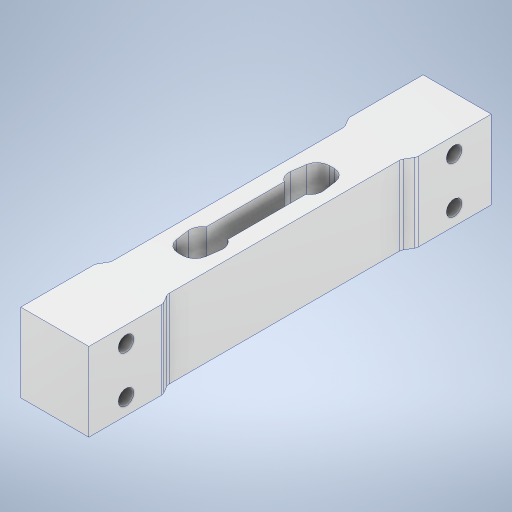
# Autodesk Inventor part: Célula de carga 3
Saved by Autodesk Inventor 2023.2 (Build 272271030, 271C)
## iProperties
Created: 2023-04-15
Part Number: Célula de carga 3
Material: Alumínio 6061
Document SubType Name: Sheet Metal
Designer: Mateus PC
Density: 2.7 g/cm^3
Sheet Metal Rule: Padrão_mm
Appearance: Alumínio - Plano
Author: Mateus PC
Autodesk Inventor part; units mm, degrees
ref_plane "YZ Plane" through (0, 0, 0) normal (1, 0, 0) x (0, 1, 0)
ref_plane "XZ Plane" through (0, 0, 0) normal (0, 1, 0) x (-1, 0, 0)
ref_plane "XY Plane" through (0, 0, 0) normal (0, 0, 1) x (1, 0, 0)
sketch "Esboço1" plane through (0, 0, 0) normal (0, 1, 0) x (-1, 0, 0)
  line L0 (0, 0) -> (22, 0)
  line L1 (22, 0) -> (22, -23.4641)
  line L2 (22, -24) -> (25.6764, -24) construction
  line L3 (0, 0) -> (0, -23.4641)
  line L4 (1.9, -27.8268) -> (1.9, -102.1732)
  line L5 (0, -106.5359) -> (0, -130)
  line L6 (0, -130) -> (22, -130)
  line L7 (22, -130) -> (22, -106.5359)
  line L8 (20.1, -102.1732) -> (20.1, -27.8268)
  line L9 (21.7321, -24.4641) -> (20.3679, -26.8268)
  line L10 (1.6321, -26.8268) -> (0.2679, -24.4641)
  line L11 (20.3679, -103.1732) -> (21.7321, -105.5359)
  line L12 (0.2679, -105.5359) -> (1.6321, -103.1732)
  arc A0 (21.7321, -24.4641) -> (22, -23.4641) centre (20, -23.4641) ccw
  arc A1 (20.3679, -26.8268) -> (20.1, -27.8268) centre (22.1, -27.8268) ccw
  arc A2 (1.9, -27.8268) -> (1.6321, -26.8268) centre (-0.1, -27.8268) ccw
  arc A3 (0, -23.4641) -> (0.2679, -24.4641) centre (2, -23.4641) ccw
  arc A4 (22, -106.5359) -> (21.7321, -105.5359) centre (20, -106.5359) ccw
  arc A5 (20.1, -102.1732) -> (20.3679, -103.1732) centre (22.1, -102.1732) ccw
  arc A6 (1.6321, -103.1732) -> (1.9, -102.1732) centre (-0.1, -102.1732) ccw
  arc A7 (0.2679, -105.5359) -> (0, -106.5359) centre (2, -106.5359) ccw
  line L13 (7.5, -52.4035) -> (7.5, -77.5965)
  spline S0 degree 3 poles (7.5, -52.4035) (7.1712, -52.2005) (6.8736, -51.9509) (6.3593, -51.374) (6.1453, -51.0498) (5.8168, -50.3503) (5.704, -49.9786) (5.5886, -49.2144) (5.5866, -48.826) (5.6404, -48.4433) knots 0 0 0 0 0.250007 0.250007 0.5 0.5 0.749993 0.749993 1 1 1 1
  line L14 (5.6404, -48.4433) -> (6.2661, -43.9914)
  spline S1 degree 3 poles (6.2661, -43.9914) (6.3326, -43.5177) (6.4837, -43.0598) (6.9401, -42.2191) (7.2419, -41.8431) (7.9639, -41.2155) (8.3783, -40.9689) (9.2743, -40.6339) (9.7488, -40.5481) (10.2271, -40.5481) knots -0.574004 -0.574004 -0.574004 -0.574004 -0.430503 -0.430503 -0.287003 -0.287003 -0.143502 -0.143502 -0.000001 -0.000001 -0.000001 -0.000001
  line L15 (10.2271, -40.5481) -> (11.7729, -40.5481)
  spline S2 degree 3 poles (11.7729, -40.5481) (12.2512, -40.5481) (12.7257, -40.6339) (13.6217, -40.9689) (14.0361, -41.2155) (14.7581, -41.8431) (15.0599, -42.2191) (15.5163, -43.0598) (15.6674, -43.5177) (15.7339, -43.9914) knots -0.574004 -0.574004 -0.574004 -0.574004 -0.430503 -0.430503 -0.287003 -0.287003 -0.143502 -0.143502 -0.000001 -0.000001 -0.000001 -0.000001
  line L16 (15.7339, -43.9914) -> (16.3596, -48.4433)
  spline S3 degree 3 poles (16.3596, -48.4433) (16.4134, -48.826) (16.4114, -49.2144) (16.296, -49.9786) (16.1832, -50.3503) (15.8547, -51.0498) (15.6407, -51.374) (15.1264, -51.9509) (14.8288, -52.2005) (14.5, -52.4035) knots 0 0 0 0 0.250007 0.250007 0.5 0.5 0.749993 0.749993 1 1 1 1
  line L17 (14.5, -77.5965) -> (14.5, -52.4035)
  spline S4 degree 3 poles (14.5, -77.5965) (14.8288, -77.7995) (15.1264, -78.0491) (15.6407, -78.626) (15.8547, -78.9502) (16.1832, -79.6497) (16.296, -80.0214) (16.4114, -80.7856) (16.4134, -81.174) (16.3596, -81.5567) knots 0 0 0 0 0.250007 0.250007 0.5 0.5 0.749993 0.749993 1 1 1 1
  line L18 (15.7339, -86.0086) -> (16.3596, -81.5567)
  spline S5 degree 3 poles (15.7339, -86.0086) (15.6674, -86.4823) (15.5163, -86.9402) (15.0599, -87.7809) (14.7581, -88.1569) (14.0361, -88.7845) (13.6217, -89.0311) (12.7257, -89.3661) (12.2512, -89.4519) (11.7729, -89.4519) knots -0.574004 -0.574004 -0.574004 -0.574004 -0.430503 -0.430503 -0.287003 -0.287003 -0.143502 -0.143502 -0.000001 -0.000001 -0.000001 -0.000001
  spline S6 degree 3 poles (10.2271, -89.4519) (9.7488, -89.4519) (9.2743, -89.3661) (8.3783, -89.0311) (7.9639, -88.7845) (7.2419, -88.1569) (6.9401, -87.7809) (6.4837, -86.9402) (6.3326, -86.4823) (6.2661, -86.0086) knots -0.574004 -0.574004 -0.574004 -0.574004 -0.430503 -0.430503 -0.287003 -0.287003 -0.143502 -0.143502 -0.000001 -0.000001 -0.000001 -0.000001
  line L19 (10.2271, -89.4519) -> (11.7729, -89.4519)
  line L20 (5.6404, -81.5567) -> (6.2661, -86.0086)
  spline S7 degree 3 poles (5.6404, -81.5567) (5.5866, -81.174) (5.5886, -80.7856) (5.704, -80.0214) (5.8168, -79.6497) (6.1453, -78.9502) (6.3593, -78.626) (6.8736, -78.0491) (7.1712, -77.7995) (7.5, -77.5965) knots 0 0 0 0 0.250007 0.250007 0.5 0.5 0.749993 0.749993 1 1 1 1
  point P0 (20.1, -27.2909)
  point P1 (0, -24)
  point P2 (1.9, -27.2909)
  point P3 (0, -106)
  point P4 (22, -106)
  point P5 (20.1, -102.7091)
  point P6 (11, -130)
  point P7 (11, -89.4519)
  point P8 (11, -40.5481)
  point P9 (20.1, -65)
  point P10 (14.5, -65)
  dimension "d0" = 22
  dimension "d1" = 24
  dimension "d4" = 3.8
  dimension "d6" = 3.8
  dimension "d7" = 24
  dimension "d8" = 18.2
  dimension "d10" = 0
  dimension "d11" = 130
  dimension "d12" = 1.9
  dimension "d13" = 2
  dimension "d14" = 2
  dimension "d38" = 7
  dimension "d39" = 7
  dimension "d40" = 4.4957
  dimension "d41" = 4.4957
  dimension "d42" = 4.4519
  dimension "d43" = 0.6257
  dimension "d44" = 172
  dimension "d45" = 1.5457
  dimension "d46" = 1.5457
  dimension "d47" = 0.6257
  dimension "d48" = 4.4519
  dimension "d49" = 3.9611
  dimension "d50" = 3.4433
  dimension "d51" = 9.4679
  dimension "d52" = 3.9611
  dimension "d53" = 3.9602
  dimension "d54" = 1.8596
  dimension "d55" = 4.4519
  dimension "d56" = 3.9602
  dimension "d57" = 3.9602
  dimension "d58" = 4.3751
  dimension "d59" = 1.8596
  dimension "d60" = 3.9611
  dimension "d61" = 3.9611
  dimension "d62" = 3.4433
  dimension "d63" = 3.4433
  dimension "d64" = 0
  dimension "d65" = 48.9038
  dimension "d67" = 0
  constraints: 42 end point, 16 point on circle, 16 point on line, 16 tangent, 8 centre point, 6 equal length, 6 equal radius, 5 midpoint, 4 horizontal, 4 vertical, 3 perpendicular, 1 parallel, 16 other
  measures "d0" distance of L0.start L0.end
  measures "d1" distance of L0.end L2.start
  measures "d4" distance of point (0, -24) point (1.9, -27.291)
  measures "d6" distance of point (22, -106) point (20.1, -102.709)
  measures "d7" distance of point (0, -106) L5.end
  measures "d8" distance between parallel lines of L4 L8
  measures "d10" vertical distance of point (1.9, -27.291) point (20.1, -27.291)
  measures "d11" distance of L6.end L0.end
  measures "d12" horizontal distance of L2.start point (20.1, -27.291)
  measures "d13" radius of A0
  measures "d14" radius of A7
  measures "d38" distance between parallel lines of L13 L17
  measures "d39" distance of L13.end L17.start
  measures "d40" distance of L16.start L16.end
  measures "d41" distance of L14.start L14.end
  measures "d42" vertical distance of L14.start L14.end
  measures "d43" horizontal distance of L14.start L14.end
  measures "d44" angle of L13 L14
  measures "d45" distance of L15.start L15.end
  measures "d46" distance of L19.start L19.end
  measures "d47" horizontal distance of L20.start L20.end
  measures "d48" vertical distance of L18.end L18.start
  measures "d49" horizontal distance of L18.start L19.end
  measures "d50" vertical distance of L19.end L18.start
  measures "d51" distance of L20.end L18.start
  measures "d52" horizontal distance of L20.end L19.start
  measures "d53" vertical distance of L20.start L13.end
  measures "d54" horizontal distance of L20.start L13.end
  measures "d55" vertical distance of L16.end L16.start
  measures "d56" vertical distance of L16.end L17.end
  measures "d57" vertical distance of L14.start L13.start
  measures "d58" distance of L13.start L14.start
  measures "d59" horizontal distance of L16.end L17.end
  measures "d60" horizontal distance of L14.end L15.start
  measures "d61" horizontal distance of L15.end L16.start
  measures "d62" vertical distance of L15.end L16.start
  measures "d63" vertical distance of L15.start L14.end
  measures "d64" horizontal distance of point (11, -89.452) point (11, -130)
  measures "d65" distance of point (11, -40.548) point (11, -89.452)
  measures "d67" vertical distance of point (14.5, -65) point (20.1, -65)
extrude "Extrusão1" add sketch "Esboço1" along normal blind 25.4
sketch "Esboço2" plane through (0, 0, 0) normal (1, 0, 0) x (0, 0, -1)
  line L0 (0, 0) -> (0, 25.4) projected
  line L1 (0, 25.4) -> (23.4641, 25.4) projected
  line L2 (130, 0) -> (130, 25.4) projected
  line L3 (106.5359, 25.4) -> (130, 25.4) projected
  point P0 (12, 20.2)
  point P1 (12, 5.2)
  point P2 (118, 20.2)
  point P3 (118, 5.2)
  point P4 (11.7321, 25.4)
  dimension "d70" = 15
  dimension "d72" = 25.4
  dimension "d73" = 5.2
  dimension "d74" = 0
  dimension "d75" = 12
  dimension "d76" = 15
  dimension "d77" = 12
  dimension "d78" = 0
  dimension "d79" = 5.2
  constraints: 1 midpoint
  measures "d70" distance of point (12, 5.2) point (12, 20.2)
  measures "d72" distance of L0.start L0.end
  measures "d73" distance from line of L1 point (12, 20.2)
  measures "d74" horizontal distance of point (12, 5.2) point (12, 20.2)
  measures "d75" distance from line of L0 point (12, 20.2)
  measures "d76" distance of point (118, 5.2) point (118, 20.2)
  measures "d77" distance from line of L2 point (118, 20.2)
  measures "d78" horizontal distance of point (118, 20.2) point (118, 5.2)
  measures "d79" distance from line of L3 point (118, 20.2)
hole "Furo1" at (0, 20.2, -12) at (0, 5.2, -12) at (0, 20.2, -118) at (0, 5.2, -118) direction (-1, 0, 0) diameter 5 end through all
equation "\"d7\" = d1"
equation "\"d12\" = -0.5 * d8 + 0.5 * d0"
equation "\"d73\" = -0.5 * d70 + 0.5 * d72"
equation "\"d76\" = d70"
equation "\"d77\" = d75"
equation "\"d79\" = d73"
equation "\"d85\" = Espessura"
equation "\"Raio_vergadura\" = Espessura"
equation "\"Largura_alívio_de_vergadura\" = Espessura"
equation "\"Profundidade_alívio_de_vergadura\" = 0.5 * Espessura"
equation "\"Tamanho_alívio_de_dobra\" = 4 * Espessura"
equation "\"Remanescente_mínimo\" = 2 * Espessura"
equation "\"Raiodetransição\" = Raio_vergadura"
equation "\"Tamanho_de_raio_de_Jacobi\" = Raio_vergadura"
equation "\"TamanhoFolga\" = Espessura"
equation "\"Espessura\" = 0.5"
